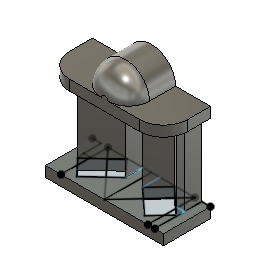
Sensorhalter_Schleifpunkt V1 (Autodesk Fusion 360 design; units mm, degrees)
Autodesk Fusion 360 part; units mm, degrees
sketch "Skizze1" plane through (0, 0, 0) normal (0, 1, 0) x (1, 0, 0)
  line L0 (0, 0) -> (0, -13.5)
  line L1 (0, -13.5) -> (34, -13.5)
  line L2 (34, -13.5) -> (34, 0)
  line L3 (34, 0) -> (0, 0)
  dimension "d1" = 13.5
  dimension "d2" = 34
  constraint coincident L0.start L3.end
  constraint vertical L0
  constraint perpendicular L0 L1
  constraint perpendicular L1 L2
  constraint perpendicular L0 L3
  measures "d1" distance of L0.start L0.end
  measures "d2" distance of L0.end L1.end
extrude "Extrusion1" add sketch "Skizze1" along normal blind 3
sketch "Skizze2" plane through (0, 3, 0) normal (0, 1, 0) x (-1, 0, 0)
  line L0 (-34, 0) -> (0, 0)
  line L1 (0, 0) -> (0, 13.5)
  line L2 (0, 13.5) -> (-34, 13.5)
  line L3 (-34, 13.5) -> (-34, 0)
  line L4 (-34, 0) -> (-31.5, 0)
  line L5 (-31.5, 0) -> (-31.5, 5)
  line L6 (-31.5, 5) -> (-29.5, 5)
  line L7 (-29.5, 5) -> (-29.5, 0)
  line L8 (0, 0) -> (-2.5, 0)
  line L9 (-2.5, 0) -> (-2.5, 5)
  line L10 (-2.5, 5) -> (-4.5, 5)
  line L11 (-4.5, 5) -> (-4.5, 0)
  line L12 (-4.5, 5) -> (-4.5, 13.5)
  line L13 (-29.5, 5) -> (-29.5, 13.5)
  line L14 (-4.5, 0) -> (-29.5, 0)
  line L15 (-4.5, 0) -> (-17, 13.5)
  line L16 (-29.5, 0) -> (-17, 13.5)
  line L17 (-25.3803, 4.4492) -> (-29.5, 0)
  line L18 (-31.5, 5) -> (-31.5, 13.5)
  line L19 (-17, 0) -> (-17, 13.5)
  line L20 (-29.5, 0) -> (-26.7824, 2.935)
  line L21 (-26.7824, 2.935) -> (-23.8473, 0.2174)
  line L22 (-26.7824, 2.935) -> (-31.1849, 7.0115)
  line L23 (-31.1849, 7.0115) -> (-26.7688, 11.7809)
  line L24 (-26.7688, 11.7809) -> (-19.4312, 4.9869)
  line L25 (-19.4312, 4.9869) -> (-23.8473, 0.2174)
  line L26 (-4.5, 0) -> (-7.2176, 2.935)
  line L27 (-7.2176, 2.935) -> (-10.1527, 0.2174)
  line L28 (-10.1527, 0.2174) -> (-7.2176, 2.935)
  line L29 (-7.2176, 2.935) -> (-2.8151, 7.0115)
  line L30 (-2.8151, 7.0115) -> (-7.2312, 11.7809)
  line L31 (-7.2312, 11.7809) -> (-14.5688, 4.9869)
  line L32 (-14.5688, 4.9869) -> (-10.1527, 0.2174)
  line L33 (-29.5, 0) -> (-29.5, 5)
  line L34 (-31.5, 5) -> (-29.5, 5)
  line L35 (-19.4312, 4.9869) -> (-19.4286, 0)
  line L36 (-14.5688, 4.9869) -> (-14.5319, 0)
  line L37 (-2.8151, 7.0115) -> (-2.5, 5)
  line L38 (-31.1849, 7.0115) -> (-31.5, 5)
  dimension "d5" = 2.5
  dimension "d6" = 2
  dimension "d7" = 2.5
  dimension "d8" = 5
  dimension "d9" = 2
  dimension "d10" = 4
  dimension "d11" = 4
  dimension "d12" = 6
  dimension "d13" = 6.5
  dimension "d14" = 10
  dimension "d15" = 4
  dimension "d16" = 4
  dimension "d17" = 6
  dimension "d18" = 6.5
  dimension "d19" = 10
  constraint coincident L0.start L3.end
  constraint perpendicular L3 L4
  constraint perpendicular L4 L5
  constraint perpendicular L5 L6
  constraint coincident L0 L7.end
  constraint perpendicular L0 L7
  constraint coincident L0.end L1.start
  constraint perpendicular L1 L8
  constraint perpendicular L0 L9
  constraint perpendicular L9 L10
  constraint coincident L0 L11.end
  constraint perpendicular L0 L11
  constraint coincident L2 L12.end
  constraint perpendicular L2 L12
  constraint coincident L2 L13.end
  constraint perpendicular L2 L13
  constraint midpoint L2 L15.end
  constraint coincident L16 L17.start
  constraint coincident L2 L18.end
  constraint perpendicular L2 L18
  constraint midpoint L14 L19.start
  constraint parallel L17 L20
  constraint perpendicular L16 L21
  constraint perpendicular L20 L22
  constraint perpendicular L22 L23
  constraint perpendicular L23 L24
  constraint perpendicular L21 L25
  constraint parallel L15 L26
  constraint perpendicular L15 L27
  constraint perpendicular L26 L29
  constraint perpendicular L29 L30
  constraint perpendicular L15 L31
  constraint coincident L14 L35.end
  constraint coincident L14 L36.end
  measures "d5" distance of L0.start L4.end
  measures "d6" distance of L5.end L6.end
  measures "d7" distance of L0.end L8.end
  measures "d8" distance of L8.end L9.end
  measures "d9" distance of L9.end L10.end
  measures "d10" distance of L7.end L20.end
  measures "d11" distance of L20.end L21.end
  measures "d12" distance of L20.end L22.end
  measures "d13" distance of L22.end L23.end
  measures "d14" distance of L23.end L24.end
  measures "d15" distance of L11.end L26.end
  measures "d16" distance of L26.end L27.end
  measures "d17" distance of L26.end L29.end
  measures "d18" distance of L29.end L30.end
  measures "d19" distance of L30.end L31.end
extrude "Extrusion2" cut sketch "Skizze2" against normal blind 10 contours L13 L16 L17 L22 L23 L24 | L16 L17 L21 L24 L25 | L13 L22 L23 | L12 L15 L29 L30 L31 | L15 L27 L28 L31 L32 | L12 L29 L30
extrude "Extrusion3" add sketch "Skizze2" along normal blind 21 contours L0 L5 L6 L7 L33 L34 | L0 L14 L16 L17 L20 L21 L25 L35 | L7 L13 L16 L17 L20 L22 L33 | L6 L13 L22 L34 L38 | L0 L14 L15 L26 L27 L28 L32 L36 | L0 L9 L10 L11 | L11 L12 L15 L26 L29 | L10 L12 L29 L37
extrude "Extrusion4" add 2 faces at (5.0509, 24, 1.7391) (28.9491, 24, 1.7391) along direction (0, 1, 0) blind 1
sketch "Skizze3" plane through (0, 0, 0) normal (0, 0, -1) x (-1, 0, 0)
  line L0 (-34, 0) -> (0, 0)
  line L1 (0, 0) -> (0, 3)
  line L2 (0, 3) -> (-2.5, 3)
  line L3 (-2.5, 3) -> (-2.5, 25)
  line L4 (-2.5, 25) -> (-14.5319, 25)
  line L5 (-14.5319, 25) -> (-14.5319, 3)
  line L6 (-14.5319, 3) -> (-19.4286, 3)
  line L7 (-19.4286, 3) -> (-19.4286, 25)
  line L8 (-19.4286, 25) -> (-31.5, 25)
  line L9 (-31.5, 25) -> (-31.5, 3)
  line L10 (-31.5, 3) -> (-34, 3)
  line L11 (-34, 3) -> (-34, 0)
  line L12 (-34, 3) -> (-34, 25)
  line L13 (-34, 25) -> (0, 25)
  line L14 (0, 25) -> (0, 28)
  line L15 (0, 28) -> (-34, 28)
  line L16 (-34, 28) -> (-34, 25)
  line L17 (-17, 28) -> (-17, 21.0656)
  circle A0 centre (-17, 28) radius 6.9344
  constraint coincident L10.end L11.start
  constraint perpendicular L10 L12
  constraint perpendicular L3 L13
  constraint perpendicular L13 L14
  constraint perpendicular L14 L15
  constraint perpendicular L13 L16
  constraint midpoint L15 L17.start
  constraint perpendicular L13 L17
  constraint coincident L17.end A0
extrude "Extrusion5" add sketch "Skizze3" against normal blind 13.5 contours L8 L13 L15 L16 A0 | L4 L13 L14 L15 A0 | L8 L13 L15 L17 A0 | L15 A0 | L4 L13 L15 L17 A0
fillet "Abrundung1" radius 6 1 edges at (17, 34.9344, 13.5)
fillet "Abrundung2" radius 4 1 edges at (0, 26.5, 13.5)
fillet "Abrundung3" radius 4 1 edges at (34, 26.5, 13.5)
delete_face "Fläche löschen1" 1 faces at (33.9819, 26, 9.8802)
delete_face "Fläche löschen2" 1 faces at (0.0181, 26, 9.8802)
fillet "Abrundung4" radius 7 1 edges at (34, 26.5, 13.5)
fillet "Abrundung5" radius 7 1 edges at (0, 26.5, 13.5)
